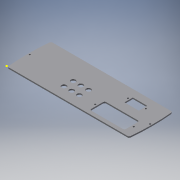
# Autodesk Inventor part: Frontplatte Apra Xdream 418
Saved by Autodesk Inventor 2018 (Build 220112000, 112)
## iProperties
Created: 2011-10-18
Part Number: Frontplatte Apra Xdream 418
Document SubType Name: Modeling
Designer: Huethe
Mass: 51.0801 g
Surface Area: 425.217 cm^2
Volume: 51.0801 cm^3
Density: 1 g/cm^3
Material: Allgemein
Appearance: Vorgabe
Author: Huethe
Autodesk Inventor part; units mm, degrees
ref_plane "YZ Plane" through (0, 0, 0) normal (1, 0, 0) x (0, 1, 0)
ref_plane "XZ Plane" through (0, 0, 0) normal (0, 1, 0) x (-1, 0, 0)
ref_plane "XY Plane" through (0, 0, 0) normal (0, 0, 1) x (1, 0, 0)
sketch "Skizze1" plane through (0, 0, 0) normal (0, 0, 1) x (1, 0, 0)
  line L0 (0, 0) -> (242, 0)
  line L1 (242, 0) -> (242, 85)
  line L2 (242, 85) -> (0, 85)
  line L3 (0, 85) -> (0, 0)
  line L4 (242, 42.5) -> (842, 42.5)
  line L5 (0, 42.5) -> (-937, 42.5)
  arc A0 (240, 0) -> (240, 85) centre (-210.5625, 42.5) ccw
  arc A1 (2, 85) -> (2, 0) centre (452.5625, 42.5) ccw
  dimension "d0" = 85
  dimension "d1" = 242
  dimension "d2" = 2
  dimension "d3" = 2
  dimension "d4" = 2
  dimension "d7" = 452.5625
  dimension "d8" = 452.5625
  constraints: 12 end point, 6 point on line, 4 point on circle, 2 centre point, 2 midpoint, 2 parallel, 2 tangent, 1 collinear, 1 horizontal, 1 perpendicular
  measures "d0" distance between parallel lines of L0 L2
  measures "d1" distance between parallel lines of L1 L3
  measures "d2" distance from line of L3 A1.start
  measures "d3" distance from line of A1.end L3
  measures "d4" distance from line of L1 A0.end
  measures "d7" radius of A0
  measures "d8" radius of A1
extrude "Extrusion1" add sketch "Skizze1" against normal blind 2.5 contours A1 L2 A0 L0
sketch "Skizze2" plane through (0, 0, 0) normal (0, 0, 1) x (1, 0, 0)
  line L0 (2, 0) -> (240, 0) projected
  line L1 (240, 85) -> (2, 85) projected
  line L2 (121, 0) -> (121, 85)
  point P0 (0, 0)
  point P1 (3.1, 42.5)
  point P2 (238.9, 42.5)
  dimension "d11" = 42.5
  dimension "d12" = 42.5
  dimension "d13" = 235.8
  dimension "d14" = 117.9
  dimension "d15" = 117.9
  constraints: 2 end point, 2 midpoint
  measures "d11" distance from line of L0 point (3.1, 42.5)
  measures "d12" distance from line of L0 point (238.9, 42.5)
  measures "d13" distance of point (238.9, 42.5) point (3.1, 42.5)
  measures "d14" distance from line of L2 point (3.1, 42.5)
  measures "d15" distance from line of L2 point (238.9, 42.5)
hole "Bohrung1" at (3.1, 42.5, 0) at (238.9, 42.5, 0) direction (0, 0, -1) diameter 3.3 depth 8 tip angle 118
sketch "Skizze3" plane through (0, 0, 0) normal (0, 0, 1) x (1, 0, 0)
  line L0 (2, 0) -> (240, 0) projected
  line L1 (240, 85) -> (2, 85) projected
  arc A0 (2, 85) -> (2, 0) centre (452.5625, 42.5) ccw projected
  line L2 (8.1386, 91.5936) -> (-1.2688, 78.1585)
  line L3 (-1.2688, 78.1585) -> (-1.2688, 91.5936)
  line L4 (-1.2688, 91.5936) -> (8.1386, 91.5936)
  line L5 (-1.7926, 7.5896) -> (9.0296, -7.8661)
  line L6 (9.0296, -7.8661) -> (-1.7926, -7.8661)
  line L7 (-1.7926, -7.8661) -> (-1.7926, 7.5896)
  line L8 (121, 0) -> (121, 85)
  line L9 (233.8614, 91.5936) -> (243.2688, 78.1585)
  line L10 (243.2688, 78.1585) -> (243.2688, 91.5936)
  line L11 (243.2688, 91.5936) -> (233.8614, 91.5936)
  line L12 (243.7926, 7.5896) -> (232.9704, -7.8661)
  line L13 (232.9704, -7.8661) -> (243.7926, -7.8661)
  line L14 (243.7926, -7.8661) -> (243.7926, 7.5896)
  point P0 (0, 0)
  point P1 (1.7712, 82.5)
  point P2 (1.7712, 2.5)
  point P3 (242, 0)
  point P4 (240.2288, 82.5)
  point P5 (240.2288, 2.5)
  dimension "d23" = 55
  dimension "d24" = 55
  dimension "d25" = 2.5
  dimension "d26" = 2.5
  constraints: 26 end point, 9 symmetric about line, 4 point on line, 3 perpendicular, 2 midpoint, 2 point on circle, 1 parallel
  measures "d23" angle of L2 L4
  measures "d24" angle of L6 L5
  measures "d25" distance from line of L0 point (1.771, 2.5)
  measures "d26" distance from line of L1 point (1.771, 82.5)
extrude "Extrusion2" cut sketch "Skizze3" against normal blind 5 contours A0 L5 L0 | L0 L5 L6 L7 A0 | L9 L11 L10 | L12 L14 L13 | L2 L3 L4 L1 A0 | A0 L1 L2
sketch "Sketch7" plane through (0, 0, 0) normal (0, 0, 1) x (1, 0, 0)
  point P0 (0, 0)
sketch "Sketch8" plane through (0, 0, 0) normal (0, 0, 1) x (1, 0, 0)
  circle A0 centre (151.8283, 22) radius 1.6
  line L0 (151.8283, 22) -> (227.3283, 22)
  circle A1 centre (227.3283, 22) radius 1.6
  line L1 (220.4783, 36.6) -> (158.6783, 36.6)
  line L2 (155.5783, 33.5) -> (155.5783, 10.5)
  line L3 (158.6783, 7.4) -> (220.4783, 7.4)
  line L4 (223.5783, 10.5) -> (223.5783, 33.5)
  line L5 (223.5783, 36.6) -> (155.5783, 7.4) construction
  line L6 (155.5783, 36.6) -> (223.5783, 7.4) construction
  arc A2 (158.6783, 36.6) -> (155.5783, 33.5) centre (158.6783, 33.5) ccw
  arc A3 (155.5783, 10.5) -> (158.6783, 7.4) centre (158.6783, 10.5) ccw
  arc A4 (220.4783, 7.4) -> (223.5783, 10.5) centre (220.4783, 10.5) ccw
  arc A5 (223.5783, 33.5) -> (220.4783, 36.6) centre (220.4783, 33.5) ccw
  line L7 (3.5217, 0) -> (238.4783, 0) projected
  line L8 (222.5783, 45) -> (177.5783, 45)
  line L9 (177.5783, 45) -> (177.5783, 61.5)
  line L10 (177.5783, 61.5) -> (222.5783, 61.5)
  line L11 (222.5783, 61.5) -> (222.5783, 45)
  line L12 (222.5783, 45) -> (177.5783, 61.5) construction
  line L13 (177.5783, 45) -> (222.5783, 61.5) construction
  line L14 (214.0783, 45) -> (186.0783, 45)
  line L15 (186.0783, 45) -> (186.0783, 61.5)
  line L16 (186.0783, 61.5) -> (214.0783, 61.5)
  line L17 (214.0783, 61.5) -> (214.0783, 45)
  line L18 (214.0783, 45) -> (186.0783, 61.5) construction
  line L19 (186.0783, 45) -> (214.0783, 61.5) construction
  circle A6 centre (217.5783, 55.5) radius 1.6
  circle A7 centre (182.5783, 55.5) radius 1.6
  arc A8 (122.7845, 17.85) -> (118.3721, 17.85) centre (120.5783, 22) ccw
  line L20 (118.3721, 17.85) -> (122.7845, 17.85)
  arc A9 (92.7845, 17.85) -> (88.3721, 17.85) centre (90.5783, 22) ccw
  line L21 (88.3721, 17.85) -> (92.7845, 17.85)
  arc A10 (107.7845, 17.85) -> (103.3721, 17.85) centre (105.5783, 22) ccw
  line L22 (103.3721, 17.85) -> (107.7845, 17.85)
  arc A11 (122.7845, 35.85) -> (118.3721, 35.85) centre (120.5783, 40) ccw
  line L23 (118.3721, 35.85) -> (122.7845, 35.85)
  line L24 (88.3721, 35.85) -> (92.7845, 35.85)
  arc A12 (92.7845, 35.85) -> (88.3721, 35.85) centre (90.5783, 40) ccw
  line L25 (103.3721, 35.85) -> (107.7845, 35.85)
  arc A13 (107.7845, 35.85) -> (103.3721, 35.85) centre (105.5783, 40) ccw
  point P0 (0, 0)
  point P1 (189.5783, 22)
  point P2 (200.0783, 53.25)
  dimension "d75" = 3.2
  dimension "d76" = 75.5
  dimension "d77" = 3.2
  dimension "d78" = 68
  dimension "d79" = 29.2
  dimension "d80" = 3.1
  dimension "d81" = 22
  dimension "d82" = 11.15
  dimension "d87" = 45
  dimension "d89" = 28
  dimension "d90" = 16.5
  dimension "d91" = 3.2
  dimension "d92" = 5
  dimension "d93" = 3.2
  dimension "d94" = 5
  dimension "d95" = 10.5
  dimension "d96" = 10.5
  dimension "d97" = 45
  dimension "d98" = 1
  dimension "d99" = 9.4
  dimension "d101" = 9.4
  dimension "d103" = 9.4
  dimension "d113" = 35
  dimension "d114" = 15
  dimension "d115" = 15
  dimension "d116" = 9.4
  dimension "d118" = 9.4
  dimension "d120" = 9.4
  dimension "d122" = 15
  dimension "d123" = 15
  dimension "d125" = 22
  dimension "d126" = 40
  dimension "d128" = 8.85
  dimension "d129" = 4.15
  constraints: 50 end point, 20 point on circle, 14 centre point, 10 horizontal, 8 point on line, 8 tangent, 7 midpoint, 6 parallel, 5 collinear, 4 horizontal alignment, 3 equal radius, 3 perpendicular, 1 coincident, 1 vertical alignment
  measures "d75" diameter of A0
  measures "d76" distance of L0.start L0.end
  measures "d77" diameter of A1
  measures "d78" distance of L6.end L5.end
  measures "d79" distance of L5.end L6.start
  measures "d80" radius of A2
  measures "d81" distance between parallel lines of L7 L0
  measures "d82" horizontal distance of L0.end L7.end
  measures "d87" distance of L9.end L10.end
  measures "d89" distance of L15.end L16.end
  measures "d90" distance of L14.end L15.end
  measures "d91" diameter of A6
  measures "d92" distance from line of L11 A6.centre
  measures "d93" diameter of A7
  measures "d94" distance from line of A7.centre L9
  measures "d95" distance from line of L8 A7.centre
  measures "d96" distance from line of L8 A6.centre
  measures "d97" distance between parallel lines of L7 L14
  measures "d98" distance between parallel lines of L4 L11
  measures "d99" diameter of A8
  measures "d101" diameter of A9
  measures "d103" diameter of A10
  measures "d113" distance from line of L2 A8.centre
  measures "d114" distance of A10.centre A8.centre
  measures "d115" distance of A9.centre A10.centre
  measures "d116" diameter of A11
  measures "d118" diameter of A12
  measures "d120" diameter of A13
  measures "d122" distance of A13.centre A11.centre
  measures "d123" distance of A12.centre A13.centre
  measures "d125" distance from line of L7 A9.centre
  measures "d126" distance from line of L7 A11.centre
  measures "d129" distance from line of A11.centre L23
extrude "Extrusion5" cut sketch "Sketch8" against normal blind 3 contours A0 | A1 | L2 A2 L1 A5 L4 L0 | L0 L4 A4 L3 A3 L2 | L8 L15 L10 L17 | A6 | A7 | L20 A8 | L21 A9 | L22 A10 | L23 A11 | A12 L24 | A13 L25
